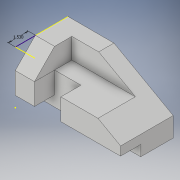
# Autodesk Inventor part: orthographic4
Saved by Autodesk Inventor 2017 (Build 210142000, 142)
## iProperties
Created: 2018-12-03
Part Number: orthographic4
Material: Generic
Document SubType Name: Modeling
Designer: qthuynh
Density: 1 g/cm^3
Appearance: Default
Author: qthuynh
Autodesk Inventor part; units mm, degrees
ref_plane "YZ Plane" through (0, 0, 0) normal (1, 0, 0) x (0, 1, 0)
ref_plane "XZ Plane" through (0, 0, 0) normal (0, 1, 0) x (-1, 0, 0)
ref_plane "XY Plane" through (0, 0, 0) normal (0, 0, 1) x (1, 0, 0)
sketch "Sketch1" plane through (0, 0, 0) normal (0, 0, 1) x (1, 0, 0)
  line L0 (0, 0) -> (203.2, 0)
  line L1 (203.2, 0) -> (203.2, 101.6)
  line L2 (203.2, 101.6) -> (0, 101.6)
  line L3 (0, 101.6) -> (0, 0)
  dimension "d0" = 203.2
  dimension "d1" = 101.6
  constraints: 8 end point, 2 parallel, 1 horizontal, 1 perpendicular
  measures "d0" distance of L2.end L1.end
  measures "d1" distance of L1.end L0.end
extrude "Extrusion1" add sketch "Sketch1" along normal blind 101.6
sketch "Sketch2" plane through (203.2, 0, 0) normal (1, 0, 0) x (0, 0, -1)
  line L0 (0, 0) -> (-101.6, 0) projected
  line L1 (-101.6, 0) -> (-62.738, 0)
  line L2 (-62.738, 0) -> (-101.6, 0)
  line L3 (-62.738, 0) -> (-62.738, 20.574)
  line L4 (-62.738, 20.574) -> (-101.6, 20.574)
  line L5 (-101.6, 0) -> (-101.6, 101.6) projected
  line L6 (-101.6, 20.574) -> (-101.6, 0)
  dimension "d4" = 38.862
  dimension "d5" = 20.574
  constraints: 10 end point, 2 collinear, 1 perpendicular, 1 point on line, 1 vertical
  measures "d4" distance of L0.end L1.end
  measures "d5" distance of L1.end L3.end
extrude "Extrusion2" cut sketch "Sketch2" against normal blind 203.2
sketch "Sketch3" plane through (0, 101.6, 0) normal (0, 1, 0) x (1, 0, 0)
  line L0 (0, 0) -> (0, -101.6) projected
  line L1 (0, -101.6) -> (37.084, -101.6)
  line L2 (203.2, -101.6) -> (0, -101.6) projected
  line L3 (37.084, -101.6) -> (37.084, -29.464)
  line L4 (37.084, -29.464) -> (159.766, -29.464)
  line L5 (159.766, -29.464) -> (159.766, -101.6)
  dimension "d8" = 37.084
  dimension "d9" = 72.136
  dimension "d10" = 122.682
  constraints: 8 end point, 3 perpendicular, 2 point on line
  measures "d8" distance of L0.end L1.end
  measures "d9" distance of L1.end L3.end
  measures "d10" distance of L3.end L4.end
sketch "Sketch4" plane through (0, 101.6, 0) normal (0, 1, 0) x (1, 0, 0)
  line L0 (203.2, -101.6) -> (0, -101.6) projected
  line L1 (37.1206, -101.6) -> (-1.7414, -101.6)
  line L2 (37.1206, -101.6) -> (37.1206, -62.738)
  line L3 (37.1206, -62.738) -> (87.9206, -62.738)
  line L4 (203.2, -62.738) -> (0, -62.738) projected
  line L5 (87.9206, -62.738) -> (87.9206, -101.6)
  point P0 (0, 0)
  dimension "d11" = 38.862
  dimension "d12" = 38.862
  dimension "d13" = 50.8
  constraints: 8 end point, 3 point on line, 1 collinear, 1 perpendicular, 1 vertical
  measures "d11" distance of L1.start L1.end
  measures "d12" distance of L1.start L2.end
  measures "d13" distance of L2.end L3.end
extrude "Extrusion3" cut sketch "Sketch4" against normal blind 203.2
extrude "Extrusion4" cut sketch "Sketch3" against normal blind 39.624
sketch "Sketch5" plane through (0, 0, 101.6) normal (0, 0, 1) x (1, 0, 0)
  line L0 (203.2, 20.574) -> (203.2, 101.6) projected
  line L1 (203.2, 101.6) -> (203.2, 37.592)
  line L2 (203.2, 37.592) -> (203.2, 101.6)
  line L3 (203.2, 101.6) -> (88.9, 101.6)
  line L4 (203.2, 101.6) -> (0, 101.6) projected
  line L5 (88.9, 101.6) -> (203.2, 37.592)
  point P0 (0, 0)
  dimension "d18" = 64.008
  dimension "d19" = 114.3
  constraints: 8 end point, 2 point on line, 1 collinear
  measures "d18" distance of L0.end L1.end
  measures "d19" distance of L0.end L3.end
extrude "Extrusion5" cut sketch "Sketch5" against normal blind 101.6
sketch "Sketch6" plane through (0, 0, 101.6) normal (0, 0, 1) x (1, 0, 0)
  point P0 (0, 0)
sketch "Sketch7" plane through (0, 101.6, 101.6) normal (0, 1, 0) x (1, 0, 0)
  line L0 (37.084, 0) -> (0, 0) projected
  line L1 (0, 0) -> (0, 38.862)
  line L2 (0, 101.6) -> (0, 0) projected
  dimension "d22" = 38.862
  constraints: 2 end point, 1 point on line
  measures "d22" distance of L0.end L1.end
sketch "Sketch8" plane through (0, 0, 0) normal (-1, 0, 0) x (0, 0, 1)
  point P0 (0, 0)
sketch "Sketch9" plane through (0, 0, 0) normal (-1, 0, 0) x (0, 0, 1)
  line L0 (101.6, 101.6) -> (101.6, 20.574) projected
  line L1 (101.6, 101.6) -> (101.6, 61.976)
  line L2 (101.6, 61.976) -> (62.8835, 101.6)
  line L3 (101.6, 101.6) -> (29.464, 101.6) projected
  line L4 (62.8835, 101.6) -> (101.6, 101.6)
  point P0 (0, 0)
  dimension "d23" = 39.624
  constraints: 6 end point, 1 collinear, 1 point on line
  measures "d23" distance of L0.start L1.end
extrude "Extrusion6" cut sketch "Sketch9" against normal blind 101.6
body "Solid1"
